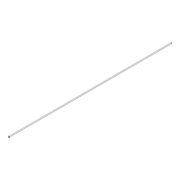
# Autodesk Inventor part: union
Saved by Autodesk Inventor 2021 (Build 250183000, 183)
## iProperties
Created: 2021-04-19
Part Number: union
Material: Genérico
Document SubType Name: Modeling
Designer: carlo
Density: 1 g/cm^3
Appearance: Valor por defecto
Author: carlo
Autodesk Inventor part; units mm, degrees
ref_plane "YZ Plane" through (0, 0, 0) normal (1, 0, 0) x (0, 1, 0)
ref_plane "XZ Plane" through (0, 0, 0) normal (0, 1, 0) x (-1, 0, 0)
ref_plane "XY Plane" through (0, 0, 0) normal (0, 0, 1) x (1, 0, 0)
sketch "Boceto1" plane through (0, 0, 0) normal (0, 0, 1) x (1, 0, 0)
  circle A0 centre (0, 0) radius 2.5
  dimension "d1" = 5
  constraints: 1 centre point, 1 coincident
  measures "d1" diameter of A0
extrude "Extrusión1" add sketch "Boceto1" along normal blind 530
